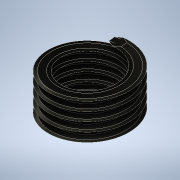
# Autodesk Inventor part: Table Decoration 2
Saved by Autodesk Inventor 2022.4 (Build 264492000, 492)
## iProperties
Created: 2024-05-02
Part Number: Table Decoration 2
Material: Generic
Document SubType Name: Modeling
Designer: t60147996
Density: 1 g/cm^3
Appearance: Gunmetal
Author: t60147996
Autodesk Inventor part; units mm, degrees
ref_plane "YZ Plane" through (0, 0, 0) normal (1, 0, 0) x (0, 1, 0)
ref_plane "XZ Plane" through (0, 0, 0) normal (0, 1, 0) x (-1, 0, 0)
ref_plane "XY Plane" through (0, 0, 0) normal (0, 0, 1) x (1, 0, 0)
sketch "Sketch1" plane through (0, 0, 0) normal (0, 1, 0) x (-1, 0, 0)
  line L0 (24.6545, -67.7063) -> (26.033, -82.3061)
  line L1 (26.033, -82.3061) -> (14.0785, -90.7998)
  line L2 (14.0785, -90.7998) -> (0.7455, -84.6937)
  line L3 (0.7455, -84.6937) -> (-0.633, -70.0939)
  line L4 (-0.633, -70.0939) -> (11.3215, -61.6002)
  line L5 (11.3215, -61.6002) -> (24.6545, -67.7063)
  point P0 (0, 0)
  point P1 (12.7, -76.2)
  point P2 (0.0562, -77.3938)
  dimension "d0" = 76.2
  dimension "d1" = 12.7
  dimension "d2" = 25.4
  constraints: 12 end point, 1 midpoint, 13 other
  measures "d0" vertical distance of point (0, 0) point (12.7, -76.2)
  measures "d1" horizontal distance of point (12.7, -76.2) point (0, 0)
  measures "d2" distance from line of point (0.056, -77.394) L0
coil "Coil1" sketch "Sketch1" operation add axis through (0, -10, 0) along (0, 1, 0) pitch 20.32 turns 5 hand right
body "Solid1"
